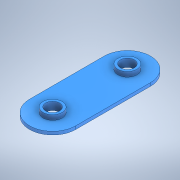
# Autodesk Inventor part: Belt_Washer
Saved by Autodesk Inventor 2021 (Build 250183000, 183)
## iProperties
Created: 2021-05-25
Part Number: Belt_Washer
Material: Generic
Document SubType Name: Modeling
Designer: Jorian Brusind
Density: 1 g/cm^3
Appearance: Cyan
Author: Jorian Brusind
Autodesk Inventor part; units mm, degrees
ref_plane "YZ Plane" through (0, 0, 0) normal (1, 0, 0) x (0, 1, 0)
ref_plane "XZ Plane" through (0, 0, 0) normal (0, 1, 0) x (-1, 0, 0)
ref_plane "XY Plane" through (0, 0, 0) normal (0, 0, 1) x (1, 0, 0)
sketch "Sketch3" plane through (0, 0, 0) normal (0, 1, 0) x (-1, 0, 0)
  line L0 (0, 0) -> (0, -47) construction
  line L1 (-14.5, 0) -> (-14.5, -47)
  line L2 (14.5, -47) -> (14.5, 0)
  arc A0 (14.5, 0) -> (-14.5, 0) centre (0, 0) ccw
  arc A1 (-14.5, -47) -> (14.5, -47) centre (0, -47) ccw
  line L3 (0, 0) -> (47, 0) construction
  circle A2 centre (0, 0) radius 4.375
  circle A3 centre (0, -47) radius 4.375
  point P0 (0, -23.5)
  dimension "d8" = 47
  dimension "d9" = 90
  dimension "d10" = 29
  dimension "d11" = 8.75
  dimension "d12" = 8.75
  constraints: 10 end point, 4 centre point, 4 point on circle, 4 tangent, 2 coincident, 1 horizontal, 1 midpoint, 1 parallel, 1 perpendicular, 1 vertical
  measures "d8" distance of L0.start L0.end
  measures "d9" angle of L0 L3
  measures "d10" diameter of A1
  measures "d11" diameter of A2
  measures "d12" diameter of A3
extrude "Extrusion3" add sketch "Sketch3" along normal blind 2
sketch "Sketch4" plane through (0, 2, 0) normal (0, 1, 0) x (1, 0, 0)
  circle A0 centre (0, 0) radius 4.375 projected
  circle A1 centre (0, 0) radius 2.75
  circle A2 centre (0, 47) radius 4.375 projected
  circle A3 centre (0, 47) radius 2.75
  circle A4 centre (0, 0) radius 6
  circle A5 centre (0, 47) radius 6
  dimension "d15" = 12
  dimension "d16" = 12
  constraints: 4 centre point, 4 coincident
  measures "d15" diameter of A4
  measures "d16" diameter of A5
extrude "Extrusion4" add sketch "Sketch4" along normal blind 3 contours A4 | A5
body "Solid2"
